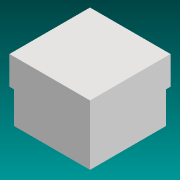
# Autodesk Inventor part: 顶盖
Saved by Autodesk Inventor 2021 (Build 250183000, 183)
## iProperties
Created: 2025-04-17
Part Number: 顶盖
Material: 常规
Document SubType Name: Modeling
Designer: 86155
Density: 1 g/cm^3
Appearance: 默认
Author: 86155
Autodesk Inventor part; units mm, degrees
ref_plane "YZ Plane" through (0, 0, 0) normal (1, 0, 0) x (0, 1, 0)
ref_plane "XZ Plane" through (0, 0, 0) normal (0, 1, 0) x (-1, 0, 0)
ref_plane "XY Plane" through (0, 0, 0) normal (0, 0, 1) x (1, 0, 0)
sketch "草图1" plane through (0, 0, 0) normal (0, 1, 0) x (-1, 0, 0)
  line L0 (0, 0) -> (-67, 0)
  line L1 (-67, 0) -> (-67, -67)
  line L2 (-67, -67) -> (0, -67)
  line L3 (0, -67) -> (0, 0)
  line L4 (-2, -2) -> (-65, -2)
  line L5 (-65, -2) -> (-65, -65)
  line L6 (-65, -65) -> (-2, -65)
  line L7 (-2, -65) -> (-2, -2)
  dimension "d0" = 67
  dimension "d1" = 67
  dimension "d2" = 2
  constraints: 16 end point, 4 parallel, 2 perpendicular, 1 horizontal, 3 other
  measures "d0" distance between parallel lines of L1 L3
  measures "d1" distance of L0.end L1.end
  measures "d2" distance between parallel lines of L3 L7
extrude "拉伸1" add sketch "草图1" along normal blind 30
sketch "草图2" plane through (0, 30, 0) normal (0, 1, 0) x (1, 0, 0)
  line L0 (67, 67) -> (0, 67) projected
  line L1 (0, 0) -> (67, 0)
  line L2 (67, 0) -> (67, 67)
  line L3 (67, 67) -> (0, 67)
  line L4 (0, 67) -> (0, 0)
  line L5 (-2, -2) -> (69, -2)
  line L6 (69, -2) -> (69, 69)
  line L7 (69, 69) -> (-2, 69)
  line L8 (-2, 69) -> (-2, -2)
  dimension "d5" = 2
  constraints: 16 end point, 4 parallel, 2 perpendicular, 1 horizontal, 3 other
  measures "d5" distance between parallel lines of L4 L8
extrude "拉伸2" add sketch "草图2" along normal blind 25 contours L2 L1 L4 L0 | L8 L7 L6 L5
fillet "圆角1" radius 3.5 4 edges at (67, 15, 0) (67, 15, -67) (0, 15, 0) (0, 15, -67)
fillet "圆角2" radius 5 8 edges at (-2, 42.5, 2) (-2, 42.5, -69) (-2, 55, -33.5) (33.5, 55, 2) (69, 42.5, 2) (69, 55, -33.5) (69, 42.5, -69) (33.5, 55, -69)
